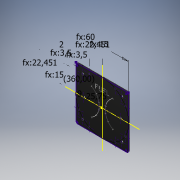
# Autodesk Inventor part: dail_face
Saved by Autodesk Inventor 2019 (Build 230136000, 136)
## iProperties
Created: 2018-04-27
Part Number: dail_face
Material: ABS Plastic
Document SubType Name: Modeling
Designer: Fierl
Density: 1.06 g/cm^3
Appearance: Smooth - White
Mass: 5.5153 g
Surface Area: 77.7264 cm^2
Volume: 5.20311 cm^3
Author: Fierl
Autodesk Inventor part; units mm, degrees
ref_plane "YZ Plane" through (0, 0, 0) normal (1, 0, 0) x (0, 1, 0)
ref_plane "XZ Plane" through (0, 0, 0) normal (0, 1, 0) x (-1, 0, 0)
ref_plane "XY Plane" through (0, 0, 0) normal (0, 0, 1) x (1, 0, 0)
sketch "Sketch1" plane through (0, 0, 0) normal (0, 0, 1) x (1, 0, 0)
  line L0 (0, -42.5799) -> (0, 42.5799) projected
  line L1 (-42.5799, 0) -> (42.5799, 0) projected
  line L2 (-28, 30) -> (28, 30)
  line L3 (30, 28) -> (30, -28)
  line L4 (28, -30) -> (-28, -30)
  line L5 (-30, -28) -> (-30, 28)
  arc A0 (-28, 30) -> (-30, 28) centre (-28, 28) ccw
  arc A1 (30, 28) -> (28, 30) centre (28, 28) ccw
  arc A2 (28, -30) -> (30, -28) centre (28, -28) ccw
  arc A3 (-30, -28) -> (-28, -30) centre (-28, -28) ccw
  point P0 (0, 0)
  point P1 (-30, 30)
  point P2 (30, 30)
  point P3 (-22.4506, 22.4506)
  point P4 (-26.5, 15)
  point P5 (-15, 26.5)
  point P6 (-15, -26.5)
  point P7 (-22.4506, -22.4506)
  point P8 (-26.5, -15)
  point P9 (26.5, -15)
  point P10 (22.4506, -22.4506)
  point P11 (15, -26.5)
  point P12 (15, 26.5)
  point P13 (22.4506, 22.4506)
  point P14 (26.5, 15)
  point P15 (-21, 0)
  point P16 (21, 0)
  point P17 (-4.25, 0)
  point P18 (4.25, 0)
  dimension "d0" = 60
  dimension "d1" = 2
  dimension "d2" = 22.4506
  dimension "d3" = 22.4506
  dimension "d4" = 15
  dimension "d5" = 15
  dimension "d6" = 3.5
  dimension "d7" = 3.5
  dimension "d10" = 360
  dimension "d28" = 9
  dimension "d36" = 25.75
  constraints: 8 end point, 8 point on circle, 8 tangent, 7 point on line, 4 centre point, 3 equal radius, 2 parallel, 2 perpendicular, 2 symmetric about line, 1 horizontal, 15 other
  measures "d0" distance of point (-30, 30) point (30, 30)
  measures "d1" radius of A0
  measures "d2" distance from line of L0 point (-22.451, 22.451)
  measures "d3" distance from line of L1 point (-22.451, 22.451)
  measures "d4" distance from line of L1 point (-26.5, 15)
  measures "d5" distance from line of L0 point (-15, 26.5)
  measures "d6" distance from line of L2 point (-15, 26.5)
  measures "d7" distance from line of L5 point (-26.5, 15)
  measures "d28" distance from line of L5 point (-21, 0)
  measures "d36" distance from line of L5 point (-4.25, 0)
extrude "Extrusion1" add sketch "Sketch1" against normal blind 1.5
hole "Hole1" at (-22.4506, 22.4506, 0) at (22.4506, 22.4506, 0) at (22.4506, -22.4506, 0) at (-22.4506, -22.4506, 0) direction (0, 0, -1) diameter 3.4 end through all clearance for "Countersunk Flat Head Screw DIN EN ISO 2009" size "M3" standard "DIN"
hole "Hole2" at (-26.5, 15, 0) at (-15, 26.5, 0) at (-15, -26.5, 0) at (-26.5, -15, 0) at (26.5, -15, 0) at (15, -26.5, 0) at (15, 26.5, 0) at (26.5, 15, 0) direction (0, 0, -1) diameter 2.4 end through all clearance for "Countersunk Flat Head Screw DIN EN ISO 2009" size "M2" standard "DIN"
hole "Hole3" at (-21, 0, 0) at (21, 0, 0) direction (0, 0, -1) diameter 3.4 end through all clearance for "Countersunk Flat Head Screw DIN EN ISO 2009" size "M3" standard "DIN"
sketch "Sketch2" plane through (0, 0, 0) normal (0, 0, 1) x (1, 0, 0)
  line L0 (21, 0) -> (36, 0) construction
  line L1 (0.1513, 29.8192) -> (0.1513, -29.8076)
  line L2 (28, 30) -> (-28, 30) projected
  arc A0 (-12, -15.5885) -> (-39, 0) centre (-21, 0) ccw construction
  arc A1 (-12.25, 15.1554) -> (-3.5031, 0.3284) centre (-21, 0) ccw construction
  line L3 (-21, 0) -> (-20.8429, 0.2721) construction
  line L4 (-21, 0) -> (-12.25, -15.1554) construction
  line L5 (-50.4, 0) -> (50.4, 0) construction
  line L6 (-12.8508, 14.6589) -> (-11.8508, 16.391)
  line L7 (-11.8508, 16.391) -> (-11.4178, 16.141)
  line L8 (-11.4178, 16.141) -> (-12.4178, 14.4089)
  line L9 (-12.4178, 14.4089) -> (-12.8508, 14.6589)
  arc A2 (-12.25, -15.1554) -> (-12.25, 15.1554) centre (-21, 0) ccw
  arc A3 (-39, 0) -> (-12, -15.5885) centre (-21, 0) ccw construction
  line L10 (-12.25, -15.1554) -> (-12, -15.5885)
  arc A4 (-12, -15.5885) -> (-12, 15.5885) centre (-21, 0) ccw
  line L11 (-12.25, -15.1554) -> (-12, -15.5885)
  arc A5 (-3.5, 0) -> (-38.5, 0) centre (-21, 0) ccw construction
  line L12 (-12.25, 15.1554) -> (-10.6363, 17.9504) construction
  line L13 (-20.8429, 0.2721) -> (-12.25, 15.1554) construction
  line L14 (-12.25, 15.1554) -> (-12, 15.5885)
  arc A6 (39.3025, 0) -> (12.3025, -15.5885) centre (21.3025, 0) ccw construction
  arc A7 (3.8056, 0.3284) -> (12.5525, 15.1554) centre (21.3025, 0) ccw construction
  line L15 (21.3025, 0) -> (12.5525, -15.1554) construction
  line L16 (50.7025, 0) -> (-50.0975, 0) construction
  arc A8 (12.5525, 15.1554) -> (12.5525, -15.1554) centre (21.3025, 0) ccw
  arc A9 (12.3025, -15.5885) -> (39.3025, 0) centre (21.3025, 0) ccw construction
  line L17 (12.5525, -15.1554) -> (12.3025, -15.5885)
  arc A10 (12.3025, 15.5885) -> (12.3025, -15.5885) centre (21.3025, 0) ccw
  line L18 (12.5525, -15.1554) -> (12.3025, -15.5885)
  arc A11 (38.8025, 0) -> (3.8025, 0) centre (21.3025, 0) ccw construction
  line L19 (12.5525, 15.1554) -> (10.9389, 17.9504) construction
  line L20 (21.1455, 0.2721) -> (12.5525, 15.1554) construction
  line L21 (12.5525, 15.1554) -> (12.3025, 15.5885)
  line L22 (-7.5931, 10.077) -> (-5.975, 11.2526)
  line L23 (-5.6811, 10.8481) -> (-7.2992, 9.6725)
  line L24 (-5.975, 11.2526) -> (-5.6811, 10.8481)
  line L25 (-7.2992, 9.6725) -> (-7.5931, 10.077)
  line L26 (-4.6534, 3.7527) -> (-2.6972, 4.1686)
  line L27 (-2.5932, 3.6795) -> (-4.5495, 3.2637)
  line L28 (-2.6972, 4.1686) -> (-2.5932, 3.6795)
  line L29 (-4.5495, 3.2637) -> (-4.6534, 3.7527)
  line L30 (-4.5403, -3.2205) -> (-2.584, -3.6363)
  line L31 (-2.688, -4.1253) -> (-4.6443, -3.7095)
  line L32 (-2.584, -3.6363) -> (-2.688, -4.1253)
  line L33 (-4.6443, -3.7095) -> (-4.5403, -3.2205)
  line L34 (-7.2732, -9.6368) -> (-5.6552, -10.8124)
  line L35 (-5.9491, -11.2169) -> (-7.5671, -10.0413)
  line L36 (-5.6552, -10.8124) -> (-5.9491, -11.2169)
  line L37 (-7.5671, -10.0413) -> (-7.2732, -9.6368)
  line L38 (-12.3796, -14.3868) -> (-11.3796, -16.1189)
  line L39 (-11.8126, -16.3689) -> (-12.8126, -14.6368)
  line L40 (-11.3796, -16.1189) -> (-11.8126, -16.3689)
  line L41 (-12.8126, -14.6368) -> (-12.3796, -14.3868)
  arc A12 (39.3025, 0) -> (12.3025, -15.5885) centre (21.3025, 0) ccw construction
  arc A13 (3.8056, 0.3284) -> (12.5525, 15.1554) centre (21.3025, 0) ccw construction
  line L42 (21.3025, 0) -> (12.5525, -15.1554) construction
  line L43 (13.1534, 14.6589) -> (12.1534, 16.391)
  line L44 (12.1534, 16.391) -> (11.7204, 16.141)
  line L45 (11.7204, 16.141) -> (12.7204, 14.4089)
  line L46 (12.7204, 14.4089) -> (13.1534, 14.6589)
  arc A14 (12.5525, 15.1554) -> (12.5525, -15.1554) centre (21.3025, 0) ccw
  arc A15 (12.3025, -15.5885) -> (39.3025, 0) centre (21.3025, 0) ccw construction
  line L47 (12.5525, -15.1554) -> (12.3025, -15.5885)
  arc A16 (12.3025, 15.5885) -> (12.3025, -15.5885) centre (21.3025, 0) ccw
  line L48 (12.5525, -15.1554) -> (12.3025, -15.5885)
  arc A17 (38.8025, 0) -> (3.8025, 0) centre (21.3025, 0) ccw construction
  line L49 (12.5525, 15.1554) -> (10.9389, 17.9504) construction
  line L50 (12.5525, 15.1554) -> (12.3025, 15.5885)
  line L51 (7.8956, 10.077) -> (6.2776, 11.2526)
  line L52 (5.9837, 10.8481) -> (7.6017, 9.6725)
  line L53 (6.2776, 11.2526) -> (5.9837, 10.8481)
  line L54 (7.6017, 9.6725) -> (7.8956, 10.077)
  line L55 (4.956, 3.7527) -> (2.9997, 4.1686)
  line L56 (2.8957, 3.6795) -> (4.852, 3.2637)
  line L57 (2.9997, 4.1686) -> (2.8957, 3.6795)
  line L58 (4.852, 3.2637) -> (4.956, 3.7527)
  line L59 (4.8429, -3.2205) -> (2.8866, -3.6363)
  line L60 (2.9905, -4.1253) -> (4.9468, -3.7095)
  line L61 (2.8866, -3.6363) -> (2.9905, -4.1253)
  line L62 (4.9468, -3.7095) -> (4.8429, -3.2205)
  line L63 (7.5757, -9.6368) -> (5.9577, -10.8124)
  line L64 (6.2516, -11.2169) -> (7.8696, -10.0413)
  line L65 (5.9577, -10.8124) -> (6.2516, -11.2169)
  line L66 (7.8696, -10.0413) -> (7.5757, -9.6368)
  line L67 (12.6821, -14.3868) -> (11.6821, -16.1189)
  line L68 (12.1151, -16.3689) -> (13.1151, -14.6368)
  line L69 (11.6821, -16.1189) -> (12.1151, -16.3689)
  line L70 (13.1151, -14.6368) -> (12.6821, -14.3868)
  line L71 (-4.899, 19.6483) -> (-7.2837, 19.6483)
  line L72 (-7.2837, 19.6483) -> (-7.2837, 18.3464)
  line L73 (-7.2837, 18.3464) -> (-5.4596, 18.3464)
  spline S0 degree 2 poles (-5.4596, 18.3464) (-5.1601, 18.3464) (-5.1601, 18.043) knots 0 0 0 1 1 1
  spline S1 degree 2 poles (-5.1601, 18.043) (-5.1601, 17.7358) (-5.4596, 17.7358) knots 0 0 0 1 1 1
  line L74 (-5.4596, 17.7358) -> (-7.2837, 17.7358)
  line L75 (-7.2837, 17.7358) -> (-7.2837, 15.6045)
  spline S2 degree 2 poles (-7.2837, 15.6045) (-7.2837, 15.2934) (-7.5756, 15.2934) knots 0 0 0 1 1 1
  spline S3 degree 2 poles (-7.5756, 15.2934) (-7.8713, 15.2934) (-7.8713, 15.6045) knots 0 0 0 1 1 1
  line L76 (-7.8713, 15.6045) -> (-7.8713, 20.2589)
  line L77 (-7.8713, 20.2589) -> (-4.899, 20.2589)
  spline S4 degree 2 poles (-4.899, 20.2589) (-4.5994, 20.2589) (-4.5994, 19.9555) knots 0 0 0 1 1 1
  spline S5 degree 2 poles (-4.5994, 19.9555) (-4.5994, 19.6483) (-4.899, 19.6483) knots 0 0 0 1 1 1
  spline S6 degree 2 poles (-0.2023, 16.9409) (-0.2023, 15.3626) (-1.8383, 15.2397) knots 0 0 0 1 1 1
  spline S7 degree 2 poles (-1.8383, 15.2397) (-2.5218, 15.1897) (-3.0595, 15.6122) knots 0 0 0 1 1 1
  spline S8 degree 2 poles (-3.0595, 15.6122) (-3.6547, 16.0845) (-3.6547, 16.8987) knots 0 0 0 1 1 1
  line L78 (-3.6547, 16.8987) -> (-3.6547, 19.9593)
  spline S9 degree 2 poles (-3.6547, 19.9593) (-3.6547, 20.2704) (-3.3552, 20.2704) knots 0 0 0 1 1 1
  spline S10 degree 2 poles (-3.3552, 20.2704) (-3.0595, 20.2704) (-3.0595, 19.9593) knots 0 0 0 1 1 1
  line L79 (-3.0595, 19.9593) -> (-3.0595, 16.8987)
  spline S11 degree 2 poles (-3.0595, 16.8987) (-3.0595, 16.3725) (-2.6755, 16.0768) knots 0 0 0 1 1 1
  spline S12 degree 2 poles (-2.6755, 16.0768) (-2.3337, 15.8119) (-1.8805, 15.8426) knots 0 0 0 1 1 1
  spline S13 degree 2 poles (-1.8805, 15.8426) (-0.7899, 15.9079) (-0.7899, 16.9409) knots 0 0 0 1 1 1
  line L80 (-0.7899, 16.9409) -> (-0.7899, 19.9593)
  spline S14 degree 2 poles (-0.7899, 19.9593) (-0.7899, 20.2704) (-0.4942, 20.2704) knots 0 0 0 1 1 1
  spline S15 degree 2 poles (-0.4942, 20.2704) (-0.2023, 20.2704) (-0.2023, 19.9593) knots 0 0 0 1 1 1
  line L81 (-0.2023, 19.9593) -> (-0.2023, 16.9409)
  line L82 (3.6302, 15.3434) -> (0.6579, 15.3434)
  line L83 (0.6579, 15.3434) -> (0.6579, 20.2627)
  line L84 (0.6579, 20.2627) -> (3.6302, 20.2627)
  spline S16 degree 2 poles (3.6302, 20.2627) (3.9298, 20.2627) (3.9298, 19.9593) knots 0 0 0 1 1 1
  spline S17 degree 2 poles (3.9298, 19.9593) (3.9298, 19.6521) (3.6302, 19.6521) knots 0 0 0 1 1 1
  line L85 (3.6302, 19.6521) -> (1.2454, 19.6521)
  line L86 (1.2454, 19.6521) -> (1.2454, 18.3464)
  line L87 (1.2454, 18.3464) -> (3.4843, 18.3464)
  spline S18 degree 2 poles (3.4843, 18.3464) (3.7838, 18.3464) (3.7838, 18.043) knots 0 0 0 1 1 1
  spline S19 degree 2 poles (3.7838, 18.043) (3.7838, 17.7358) (3.4843, 17.7358) knots 0 0 0 1 1 1
  line L88 (3.4843, 17.7358) -> (1.2454, 17.7358)
  line L89 (1.2454, 17.7358) -> (1.2454, 15.954)
  line L90 (1.2454, 15.954) -> (3.6302, 15.954)
  spline S20 degree 2 poles (3.6302, 15.954) (3.9298, 15.954) (3.9298, 15.6506) knots 0 0 0 1 1 1
  spline S21 degree 2 poles (3.9298, 15.6506) (3.9298, 15.3434) (3.6302, 15.3434) knots 0 0 0 1 1 1
  line L91 (7.962, 15.3357) -> (4.9897, 15.3357)
  line L92 (4.9897, 15.3357) -> (4.9897, 19.9516)
  spline S22 degree 2 poles (4.9897, 19.9516) (4.9897, 20.2627) (5.2854, 20.2627) knots 0 0 0 1 1 1
  spline S23 degree 2 poles (5.2854, 20.2627) (5.5772, 20.2627) (5.5772, 19.9516) knots 0 0 0 1 1 1
  line L93 (5.5772, 19.9516) -> (5.5772, 15.9386)
  line L94 (5.5772, 15.9386) -> (7.962, 15.9386)
  spline S24 degree 2 poles (7.962, 15.9386) (8.2616, 15.9386) (8.2616, 15.6391) knots 0 0 0 1 1 1
  spline S25 degree 2 poles (8.2616, 15.6391) (8.2616, 15.3357) (7.962, 15.3357) knots 0 0 0 1 1 1
  point P0 (0, 0)
  point P1 (21, 0)
  point P2 (21, 0)
  point P3 (-8.2822, 20.2704)
  dimension "encoder_extrude_hight" = 3
  dimension "d69" = 36
  dimension "d70" = 35
  dimension "d71" = 120
  dimension "d72" = 2
  dimension "d73" = 0.5
  dimension "d78" = 18
  dimension "d79" = 17.5
  dimension "d82" = 120
  constraints: 139 end point, 45 symmetric about line, 42 point on circle, 18 centre point, 9 coincident, 4 point on line, 2 parallel, 1 horizontal, 1 perpendicular, 1 vertical, 60 other
  measures "d69" diameter of A0
  measures "d70" diameter of A1
  measures "d71" angle of L4 L3
  measures "d72" distance of L7.end L8.end
  measures "d73" distance of L6.end L7.end
  measures "d78" radius of A4
  measures "d79" radius of A2
extrude "Extrusion2" cut sketch "Sketch2" against normal blind 0.1
equation "\"d0\" = backplate_width"
equation "\"d2\" = hole_distance"
equation "\"d3\" = hole_distance"
equation "\"d4\" = screw_distance_center"
equation "\"d5\" = screw_distance_center"
equation "\"d6\" = screw_distance_outside"
equation "\"d7\" = screw_distance_outside"
equation "\"encoder_extrude_hight\" = 3"
equation "\"encoder_axis\" = 8"
equation "\"encoder_emboss\" = 0"
equation "\"encoders\" = 0"
equation "\"encoder_width\" = 27"
equation "\"front_plate_thickness\" = 2"
equation "\"glass_thickness\" = 2"
equation "\"screw_distance_outside\" = 3.5"
equation "\"encoder_rad\" = 49"
equation "\"screw_distance_center\" = 15"
equation "\"ring_top_thickness\" = 2"
equation "\"ring_outer_bevel_depth\" = 0.5"
equation "\"ring_depth\" = 6"
equation "\"ring_outer_bevel_height\" = 3"
equation "\"ring_inner_bevel_depth\" = 3.5"
equation "\"ring_thickness\" = 9"
equation "\"hole_from_center\" = 63.5"
equation "\"circle_dimension_inner\" = 47"
equation "\"circle_dimension\" = 56"
equation "\"backplate_width\" = 60"
equation "\"hole_distance\" = 22.45064"
body "Solid1"
